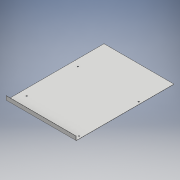
# Autodesk Inventor part: dads trunk
Saved by Autodesk Inventor 2018 (Build 220112000, 112)
## iProperties
Created: 2018-06-19
Part Number: dads trunk
Material: Generic
Document SubType Name: Sheet Metal
Designer: John Viljoen
Density: 1 g/cm^3
Flat Pattern Width: 18.1174 cm
Flat Pattern Length: 26.3586 cm
Flat Pattern Area: 477.549 cm^2
Sheet Metal Rule: Default_mm
Sheet Metal Width: 181.174 mm
Sheet Metal Length: 263.586 mm
Sheet Metal Area: 47754.925 mm^2
Appearance: Default
Author: John Viljoen
Autodesk Inventor part; units mm, degrees
ref_plane "YZ Plane" through (0, 0, 0) normal (1, 0, 0) x (0, 1, 0)
ref_plane "XZ Plane" through (0, 0, 0) normal (0, 1, 0) x (-1, 0, 0)
ref_plane "XY Plane" through (0, 0, 0) normal (0, 0, 1) x (1, 0, 0)
sketch "Sketch1" plane through (0, 0, 0) normal (0, 0, 1) x (1, 0, 0)
  line L0 (0, 0) -> (181.174, 0)
  line L1 (181.174, 0) -> (181.174, 253.26)
  line L2 (181.174, 253.26) -> (0, 253.26)
  line L3 (0, 253.26) -> (0, 0)
  dimension "d0" = 181.174
  dimension "d1" = 253.26
  measures "d0" distance of L2.end L1.end
  measures "d1" distance of L1.end L0.end
extrude "Plate1" add sketch "Sketch1" along normal blind 0.5
sketch "Sketch2" plane through (181.174, 0, 0.5) normal (0, -1, 0) x (1, 0, 0)
  line L0 (-181.174, 0) -> (0, 0)
  line L1 (0, 0) -> (0, 10.195)
  line L2 (0, 10.195) -> (-181.174, 10.195)
  line L3 (-181.174, 10.195) -> (-181.174, 0)
  constraints: 6 end point, 1 horizontal, 1 perpendicular, 1 vertical
edge flange "Flange1" height 10.695 angle 90 thickness 0.5 bend radius 0.5 thickness toward (0, -1, 0) relief straight relief width 0.5 relief depth 0.25 edges at (90.587, 0, 0.5) wall of the first edge with corners at (0, 0, 0.5) (181.174, 0, 0.5) (181.174, 0, 10.695) (0, 0, 10.695)
bend "Bend1"
corner "Corner1"
sketch "Sketch3" plane through (0, 0, 0.5) normal (0, 0, 1) x (1, 0, 0)
  line L0 (181.174, 253.26) -> (181.174, 0.5) projected
  line L1 (181.174, 253.26) -> (181.174, 168.36) construction
  line L2 (181.174, 168.36) -> (174.824, 168.36) construction
  line L3 (174.824, 168.36) -> (17.344, 168.36) construction
  line L4 (174.824, 168.36) -> (174.824, 13.48) construction
  circle A0 centre (174.824, 13.48) radius 1.5
  circle A1 centre (174.824, 168.36) radius 1.5
  circle A2 centre (17.344, 168.36) radius 1.5
  point P0 (0, 0)
  dimension "d13" = 84.9
  dimension "d14" = 6.35
  dimension "d15" = 157.48
  dimension "d16" = 154.88
  dimension "d17" = 3
  dimension "d18" = 3
  dimension "d19" = 3
  constraints: 8 end point, 3 centre point, 3 coincident, 1 horizontal, 1 perpendicular, 1 point on line, 1 vertical
  measures "d13" distance of L0.start L1.end
  measures "d14" distance of L1.end L2.end
  measures "d15" distance of L2.end L3.end
  measures "d16" distance of L2.end L4.end
  measures "d17" diameter of A0
  measures "d18" diameter of A1
  measures "d19" diameter of A2
extrude "Extrusion1" cut sketch "Sketch3" against normal blind 10
sketch "Sketch5" plane through (0, 0, 0.5) normal (0, 0, 1) x (1, 0, 0)
  circle A0 centre (17.344, 168.36) radius 1.5 projected
  line L0 (17.344, 168.36) -> (17.344, 35.808) construction
  line L1 (17.344, 168.36) -> (149.896, 168.36) construction
  circle A1 centre (17.344, 35.808) radius 1.5
  point P0 (0, 0)
  dimension "d28" = 90
  dimension "d29" = 3
  constraints: 4 end point, 1 centre point, 1 coincident, 1 horizontal, 1 perpendicular
  measures "d28" angle of L0 L1
  measures "d29" diameter of A1
extrude "Extrusion3" cut sketch "Sketch5" against normal blind 10 contours A1
equation "\"d2\" = Thickness"
equation "\"d3\" = BendReliefWidth"
equation "\"d4\" = BendReliefDepth"
equation "\"d5\" = MinimumRemnant"
equation "\"d6\" = TransitionRadius"
equation "\"d9\" = BendRadius"
equation "\"d10\" = CornerReliefSize"
equation "\"d11\" = GapSize"
equation "\"d12\" = JacobiRadiusSize"
equation "\"BendRadius\" = Thickness"
equation "\"BendReliefWidth\" = Thickness"
equation "\"BendReliefDepth\" = 0.5 * Thickness"
equation "\"CornerReliefSize\" = 4 * Thickness"
equation "\"MinimumRemnant\" = 2 * Thickness"
equation "\"TransitionRadius\" = BendRadius"
equation "\"JacobiRadiusSize\" = BendRadius"
equation "\"GapSize\" = Thickness"
equation "\"Thickness\" = 0.5"
body "Solid1"
